Autodesk Inventor part; units mm, degrees
(part 2 of 2)
  line L943 (178.544, 73.9331) -> (164.545, 73.9331)
  line L944 (145.495, 73.9331) -> (145.495, 72.9326)
  line L945 (145.495, 72.9326) -> (144.694, 72.9326)
  line L946 (144.694, 72.9326) -> (144.694, 69.8334)
  line L947 (144.694, 69.8334) -> (145.495, 69.8334)
  line L948 (145.495, 69.8334) -> (145.495, 64.0334)
  line L949 (145.495, 64.0334) -> (144.694, 64.0334)
  line L950 (144.694, 64.0334) -> (144.694, 60.9328)
  line L951 (144.694, 60.9328) -> (145.495, 60.9328)
  line L952 (145.495, 60.9328) -> (145.495, 59.9338)
  line L953 (145.495, 59.9338) -> (159.494, 59.9338)
  line L954 (159.494, 59.9338) -> (159.494, 60.9328)
  line L955 (159.494, 60.9328) -> (160.295, 60.9328)
  line L956 (160.295, 60.9328) -> (160.295, 64.0334)
  line L957 (160.295, 64.0334) -> (159.494, 64.0334)
  line L958 (159.494, 64.0334) -> (159.494, 69.8334)
  line L959 (159.494, 69.8334) -> (160.295, 69.8334)
  line L960 (160.295, 69.8334) -> (160.295, 72.9326)
  line L961 (160.295, 72.9326) -> (159.494, 72.9326)
  line L962 (159.494, 72.9326) -> (159.494, 73.9331)
  line L963 (159.494, 73.9331) -> (145.495, 73.9331)
  line L964 (126.445, 73.9331) -> (126.445, 72.9326)
  line L965 (126.445, 72.9326) -> (125.644, 72.9326)
  line L966 (125.644, 72.9326) -> (125.644, 69.8334)
  line L967 (125.644, 69.8334) -> (126.445, 69.8334)
  line L968 (126.445, 69.8334) -> (126.445, 64.0334)
  line L969 (126.445, 64.0334) -> (125.644, 64.0334)
  line L970 (125.644, 64.0334) -> (125.644, 60.9328)
  line L971 (125.644, 60.9328) -> (126.445, 60.9328)
  line L972 (126.445, 60.9328) -> (126.445, 59.9338)
  line L973 (126.445, 59.9338) -> (140.444, 59.9338)
  line L974 (140.444, 59.9338) -> (140.444, 60.9328)
  line L975 (140.444, 60.9328) -> (141.245, 60.9328)
  line L976 (141.245, 60.9328) -> (141.245, 64.0334)
  line L977 (141.245, 64.0334) -> (140.444, 64.0334)
  line L978 (140.444, 64.0334) -> (140.444, 69.8334)
  line L979 (140.444, 69.8334) -> (141.245, 69.8334)
  line L980 (141.245, 69.8334) -> (141.245, 72.9326)
  line L981 (141.245, 72.9326) -> (140.444, 72.9326)
  line L982 (140.444, 72.9326) -> (140.444, 73.9331)
  line L983 (140.444, 73.9331) -> (126.445, 73.9331)
  line L984 (107.395, 73.9331) -> (107.395, 72.9326)
  line L985 (107.395, 72.9326) -> (106.594, 72.9326)
  line L986 (106.594, 72.9326) -> (106.594, 69.8334)
  line L987 (106.594, 69.8334) -> (107.395, 69.8334)
  line L988 (107.395, 69.8334) -> (107.395, 64.0334)
  line L989 (107.395, 64.0334) -> (106.594, 64.0334)
  line L990 (106.594, 64.0334) -> (106.594, 60.9328)
  line L991 (106.594, 60.9328) -> (107.395, 60.9328)
  line L992 (107.395, 60.9328) -> (107.395, 59.9338)
  line L993 (107.395, 59.9338) -> (121.394, 59.9338)
  line L994 (121.394, 59.9338) -> (121.394, 60.9328)
  line L995 (121.394, 60.9328) -> (122.195, 60.9328)
  line L996 (122.195, 60.9328) -> (122.195, 64.0334)
  line L997 (122.195, 64.0334) -> (121.394, 64.0334)
  line L998 (121.394, 64.0334) -> (121.394, 69.8334)
  line L999 (121.394, 69.8334) -> (122.195, 69.8334)
  line L1000 (122.195, 69.8334) -> (122.195, 72.9326)
  line L1001 (122.195, 72.9326) -> (121.394, 72.9326)
  line L1002 (121.394, 72.9326) -> (121.394, 73.9331)
  line L1003 (121.394, 73.9331) -> (107.395, 73.9331)
  line L1004 (88.3447, 73.9331) -> (88.3447, 72.9326)
  line L1005 (88.3447, 72.9326) -> (87.5439, 72.9326)
  line L1006 (87.5439, 72.9326) -> (87.5439, 69.8334)
  line L1007 (87.5439, 69.8334) -> (88.3447, 69.8334)
  line L1008 (88.3447, 69.8334) -> (88.3447, 64.0334)
  line L1009 (88.3447, 64.0334) -> (87.5439, 64.0334)
  line L1010 (87.5439, 64.0334) -> (87.5439, 60.9328)
  line L1011 (87.5439, 60.9328) -> (88.3447, 60.9328)
  line L1012 (88.3447, 60.9328) -> (88.3447, 59.9338)
  line L1013 (88.3447, 59.9338) -> (102.344, 59.9338)
  line L1014 (102.344, 59.9338) -> (102.344, 60.9328)
  line L1015 (102.344, 60.9328) -> (103.145, 60.9328)
  line L1016 (103.145, 60.9328) -> (103.145, 64.0334)
  line L1017 (103.145, 64.0334) -> (102.344, 64.0334)
  line L1018 (102.344, 64.0334) -> (102.344, 69.8334)
  line L1019 (102.344, 69.8334) -> (103.145, 69.8334)
  line L1020 (103.145, 69.8334) -> (103.145, 72.9326)
  line L1021 (103.145, 72.9326) -> (102.344, 72.9326)
  line L1022 (102.344, 72.9326) -> (102.344, 73.9331)
  line L1023 (102.344, 73.9331) -> (88.3447, 73.9331)
  line L1024 (69.2947, 73.9331) -> (69.2947, 72.9326)
  line L1025 (69.2947, 72.9326) -> (68.4939, 72.9326)
  line L1026 (68.4939, 72.9326) -> (68.4939, 69.8334)
  line L1027 (68.4939, 69.8334) -> (69.2947, 69.8334)
  line L1028 (69.2947, 69.8334) -> (69.2947, 64.0334)
  line L1029 (69.2947, 64.0334) -> (68.4939, 64.0334)
  line L1030 (68.4939, 64.0334) -> (68.4939, 60.9328)
  line L1031 (68.4939, 60.9328) -> (69.2947, 60.9328)
  line L1032 (69.2947, 60.9328) -> (69.2947, 59.9338)
  line L1033 (69.2947, 59.9338) -> (83.294, 59.9338)
  line L1034 (83.294, 59.9338) -> (83.294, 60.9328)
  line L1035 (83.294, 60.9328) -> (84.0948, 60.9328)
  line L1036 (84.0948, 60.9328) -> (84.0948, 64.0334)
  line L1037 (84.0948, 64.0334) -> (83.294, 64.0334)
  line L1038 (83.294, 64.0334) -> (83.294, 69.8334)
  line L1039 (83.294, 69.8334) -> (84.0948, 69.8334)
  line L1040 (84.0948, 69.8334) -> (84.0948, 72.9326)
  line L1041 (84.0948, 72.9326) -> (83.294, 72.9326)
  line L1042 (83.294, 72.9326) -> (83.294, 73.9331)
  line L1043 (83.294, 73.9331) -> (69.2947, 73.9331)
  line L1044 (50.2447, 73.9331) -> (50.2447, 72.9326)
  line L1045 (50.2447, 72.9326) -> (49.4439, 72.9326)
  line L1046 (49.4439, 72.9326) -> (49.4439, 69.8334)
  line L1047 (49.4439, 69.8334) -> (50.2447, 69.8334)
  line L1048 (50.2447, 69.8334) -> (50.2447, 64.0334)
  line L1049 (50.2447, 64.0334) -> (49.4439, 64.0334)
  line L1050 (49.4439, 64.0334) -> (49.4439, 60.9328)
  line L1051 (49.4439, 60.9328) -> (50.2447, 60.9328)
  line L1052 (50.2447, 60.9328) -> (50.2447, 59.9338)
  line L1053 (50.2447, 59.9338) -> (64.244, 59.9338)
  line L1054 (64.244, 59.9338) -> (64.244, 60.9328)
  line L1055 (64.244, 60.9328) -> (65.0448, 60.9328)
  line L1056 (65.0448, 60.9328) -> (65.0448, 64.0334)
  line L1057 (65.0448, 64.0334) -> (64.244, 64.0334)
  line L1058 (64.244, 64.0334) -> (64.244, 69.8334)
  line L1059 (64.244, 69.8334) -> (65.0448, 69.8334)
  line L1060 (65.0448, 69.8334) -> (65.0448, 72.9326)
  line L1061 (65.0448, 72.9326) -> (64.244, 72.9326)
  line L1062 (64.244, 72.9326) -> (64.244, 73.9331)
  line L1063 (64.244, 73.9331) -> (50.2447, 73.9331)
  line L1064 (31.1947, 73.9331) -> (31.1947, 72.9326)
  line L1065 (31.1947, 72.9326) -> (30.394, 72.9326)
  line L1066 (30.394, 72.9326) -> (30.394, 69.8334)
  line L1067 (30.394, 69.8334) -> (31.1947, 69.8334)
  line L1068 (31.1947, 69.8334) -> (31.1947, 64.0334)
  line L1069 (31.1947, 64.0334) -> (30.394, 64.0334)
  line L1070 (30.394, 64.0334) -> (30.394, 60.9328)
  line L1071 (30.394, 60.9328) -> (31.1947, 60.9328)
  line L1072 (31.1947, 60.9328) -> (31.1947, 59.9338)
  line L1073 (31.1947, 59.9338) -> (45.194, 59.9338)
  line L1074 (45.194, 59.9338) -> (45.194, 60.9328)
  line L1075 (45.194, 60.9328) -> (45.9948, 60.9328)
  line L1076 (45.9948, 60.9328) -> (45.9948, 64.0334)
  line L1077 (45.9948, 64.0334) -> (45.194, 64.0334)
  line L1078 (45.194, 64.0334) -> (45.194, 69.8334)
  line L1079 (45.194, 69.8334) -> (45.9948, 69.8334)
  line L1080 (45.9948, 69.8334) -> (45.9948, 72.9326)
  line L1081 (45.9948, 72.9326) -> (45.194, 72.9326)
  line L1082 (45.194, 72.9326) -> (45.194, 73.9331)
  line L1083 (45.194, 73.9331) -> (31.1947, 73.9331)
  line L1084 (7.3822, 73.9331) -> (7.3822, 72.9326)
  line L1085 (7.3822, 72.9326) -> (6.5815, 72.9326)
  line L1086 (6.5815, 72.9326) -> (6.5815, 69.8334)
  line L1087 (6.5815, 69.8334) -> (7.3822, 69.8334)
  line L1088 (7.3822, 69.8334) -> (7.3822, 64.0334)
  line L1089 (7.3822, 64.0334) -> (6.5815, 64.0334)
  line L1090 (6.5815, 64.0334) -> (6.5815, 60.9328)
  line L1091 (6.5815, 60.9328) -> (7.3822, 60.9328)
  line L1092 (7.3822, 60.9328) -> (7.3822, 59.9338)
  line L1093 (7.3822, 59.9338) -> (21.3817, 59.9338)
  line L1094 (21.3817, 59.9338) -> (21.3817, 60.9328)
  line L1095 (21.3817, 60.9328) -> (22.1809, 60.9328)
  line L1096 (22.1809, 60.9328) -> (22.1809, 64.0334)
  line L1097 (22.1809, 64.0334) -> (21.3817, 64.0334)
  line L1098 (21.3817, 64.0334) -> (21.3817, 69.8334)
  line L1099 (21.3817, 69.8334) -> (22.1809, 69.8334)
  line L1100 (22.1809, 69.8334) -> (22.1809, 72.9326)
  line L1101 (22.1809, 72.9326) -> (21.3817, 72.9326)
  line L1102 (21.3817, 72.9326) -> (21.3817, 73.9331)
  line L1103 (21.3817, 73.9331) -> (7.3822, 73.9331)
  line L1104 (259.795, 92.9831) -> (259.795, 91.9826)
  line L1105 (259.795, 91.9826) -> (258.994, 91.9826)
  line L1106 (258.994, 91.9826) -> (258.994, 88.8834)
  line L1107 (258.994, 88.8834) -> (259.795, 88.8834)
  line L1108 (259.795, 88.8834) -> (259.795, 88.2826)
  line L1109 (259.795, 88.2826) -> (258.269, 88.2826)
  line L1110 (258.269, 88.2826) -> (258.269, 91.5127)
  line L1111 (258.269, 91.5127) -> (256.544, 91.5127)
  line L1112 (256.544, 91.5127) -> (256.544, 92.4348)
  line L1113 (256.544, 92.4348) -> (253.243, 92.4348)
  line L1114 (253.243, 92.4348) -> (253.243, 91.5127)
  line L1115 (253.243, 91.5127) -> (251.52, 91.5127)
  line L1116 (251.52, 91.5127) -> (251.52, 88.2826)
  line L1117 (251.52, 88.2826) -> (250.694, 88.2826)
  line L1118 (250.694, 88.2826) -> (250.694, 85.4837)
  line L1119 (250.694, 85.4837) -> (251.52, 85.4837)
  line L1120 (251.52, 85.4837) -> (251.52, 79.2138)
  line L1121 (251.52, 79.2138) -> (253.243, 79.2138)
  line L1122 (253.243, 79.2138) -> (253.243, 78.2327)
  line L1123 (253.243, 78.2327) -> (256.544, 78.2327)
  line L1124 (256.544, 78.2327) -> (256.544, 79.2138)
  line L1125 (256.544, 79.2138) -> (258.269, 79.2138)
  line L1126 (258.269, 79.2138) -> (258.269, 83.6828)
  line L1127 (258.269, 83.6828) -> (259.795, 83.6828)
  line L1128 (259.795, 83.6828) -> (259.795, 83.0834)
  line L1129 (259.795, 83.0834) -> (258.994, 83.0834)
  line L1130 (258.994, 83.0834) -> (258.994, 79.9828)
  line L1131 (258.994, 79.9828) -> (259.795, 79.9828)
  line L1132 (259.795, 79.9828) -> (259.795, 78.9838)
  line L1133 (259.795, 78.9838) -> (273.794, 78.9838)
  line L1134 (273.794, 78.9838) -> (273.794, 79.9828)
  line L1135 (273.794, 79.9828) -> (274.595, 79.9828)
  line L1136 (274.595, 79.9828) -> (274.595, 83.0834)
  line L1137 (274.595, 83.0834) -> (273.794, 83.0834)
  line L1138 (273.794, 83.0834) -> (273.794, 83.6828)
  line L1139 (273.794, 83.6828) -> (275.32, 83.6828)
  line L1140 (275.32, 83.6828) -> (275.32, 79.2138)
  line L1141 (275.32, 79.2138) -> (277.045, 79.2138)
  line L1142 (277.045, 79.2138) -> (277.045, 78.2327)
  line L1143 (277.045, 78.2327) -> (280.344, 78.2327)
  line L1144 (280.344, 78.2327) -> (280.344, 79.2138)
  line L1145 (280.344, 79.2138) -> (282.069, 79.2138)
  line L1146 (282.069, 79.2138) -> (282.069, 85.4837)
  line L1147 (282.069, 85.4837) -> (282.895, 85.4837)
  line L1148 (282.895, 85.4837) -> (282.895, 88.2826)
  line L1149 (282.895, 88.2826) -> (282.069, 88.2826)
  line L1150 (282.069, 88.2826) -> (282.069, 91.5127)
  line L1151 (282.069, 91.5127) -> (280.344, 91.5127)
  line L1152 (280.344, 91.5127) -> (280.344, 92.4348)
  line L1153 (280.344, 92.4348) -> (277.045, 92.4348)
  line L1154 (277.045, 92.4348) -> (277.045, 91.5127)
  line L1155 (277.045, 91.5127) -> (275.32, 91.5127)
  line L1156 (275.32, 91.5127) -> (275.32, 88.2826)
  line L1157 (275.32, 88.2826) -> (273.794, 88.2826)
  line L1158 (273.794, 88.2826) -> (273.794, 88.8834)
  line L1159 (273.794, 88.8834) -> (274.595, 88.8834)
  line L1160 (274.595, 88.8834) -> (274.595, 91.9826)
  line L1161 (274.595, 91.9826) -> (273.794, 91.9826)
  line L1162 (273.794, 91.9826) -> (273.794, 92.9831)
  line L1163 (273.794, 92.9831) -> (259.795, 92.9831)
  line L1164 (231.22, 92.9831) -> (231.22, 91.9826)
  line L1165 (231.22, 91.9826) -> (230.419, 91.9826)
  line L1166 (230.419, 91.9826) -> (230.419, 88.8834)
  line L1167 (230.419, 88.8834) -> (231.22, 88.8834)
  line L1168 (231.22, 88.8834) -> (231.22, 83.0834)
  line L1169 (231.22, 83.0834) -> (230.419, 83.0834)
  line L1170 (230.419, 83.0834) -> (230.419, 79.9828)
  line L1171 (230.419, 79.9828) -> (231.22, 79.9828)
  line L1172 (231.22, 79.9828) -> (231.22, 78.9838)
  line L1173 (231.22, 78.9838) -> (245.219, 78.9838)
  line L1174 (245.219, 78.9838) -> (245.219, 79.9828)
  line L1175 (245.219, 79.9828) -> (246.02, 79.9828)
  line L1176 (246.02, 79.9828) -> (246.02, 83.0834)
  line L1177 (246.02, 83.0834) -> (245.219, 83.0834)
  line L1178 (245.219, 83.0834) -> (245.219, 88.8834)
  line L1179 (245.219, 88.8834) -> (246.02, 88.8834)
  line L1180 (246.02, 88.8834) -> (246.02, 91.9826)
  line L1181 (246.02, 91.9826) -> (245.219, 91.9826)
  line L1182 (245.219, 91.9826) -> (245.219, 92.9831)
  line L1183 (245.219, 92.9831) -> (231.22, 92.9831)
  line L1184 (212.17, 92.9831) -> (212.17, 91.9826)
  line L1185 (212.17, 91.9826) -> (211.369, 91.9826)
  line L1186 (211.369, 91.9826) -> (211.369, 88.8834)
  line L1187 (211.369, 88.8834) -> (212.17, 88.8834)
  line L1188 (212.17, 88.8834) -> (212.17, 83.0834)
  line L1189 (212.17, 83.0834) -> (211.369, 83.0834)
  line L1190 (211.369, 83.0834) -> (211.369, 79.9828)
  line L1191 (211.369, 79.9828) -> (212.17, 79.9828)
  line L1192 (212.17, 79.9828) -> (212.17, 78.9838)
  line L1193 (212.17, 78.9838) -> (226.169, 78.9838)
  line L1194 (226.169, 78.9838) -> (226.169, 79.9828)
  line L1195 (226.169, 79.9828) -> (226.97, 79.9828)
  line L1196 (226.97, 79.9828) -> (226.97, 83.0834)
  line L1197 (226.97, 83.0834) -> (226.169, 83.0834)
  line L1198 (226.169, 83.0834) -> (226.169, 88.8834)
  line L1199 (226.169, 88.8834) -> (226.97, 88.8834)
  line L1200 (226.97, 88.8834) -> (226.97, 91.9826)
  line L1201 (226.97, 91.9826) -> (226.169, 91.9826)
  line L1202 (226.169, 91.9826) -> (226.169, 92.9831)
  line L1203 (226.169, 92.9831) -> (212.17, 92.9831)
  line L1204 (193.12, 92.9831) -> (193.12, 91.9826)
  line L1205 (193.12, 91.9826) -> (192.319, 91.9826)
  line L1206 (192.319, 91.9826) -> (192.319, 88.8834)
  line L1207 (192.319, 88.8834) -> (193.12, 88.8834)
  line L1208 (193.12, 88.8834) -> (193.12, 83.0834)
  line L1209 (193.12, 83.0834) -> (192.319, 83.0834)
  line L1210 (192.319, 83.0834) -> (192.319, 79.9828)
  line L1211 (192.319, 79.9828) -> (193.12, 79.9828)
  line L1212 (193.12, 79.9828) -> (193.12, 78.9838)
  line L1213 (193.12, 78.9838) -> (207.119, 78.9838)
  line L1214 (207.119, 78.9838) -> (207.119, 79.9828)
  line L1215 (207.119, 79.9828) -> (207.92, 79.9828)
  line L1216 (207.92, 79.9828) -> (207.92, 83.0834)
  line L1217 (207.92, 83.0834) -> (207.119, 83.0834)
  line L1218 (207.119, 83.0834) -> (207.119, 88.8834)
  line L1219 (207.119, 88.8834) -> (207.92, 88.8834)
  line L1220 (207.92, 88.8834) -> (207.92, 91.9826)
  line L1221 (207.92, 91.9826) -> (207.119, 91.9826)
  line L1222 (207.119, 91.9826) -> (207.119, 92.9831)
  line L1223 (207.119, 92.9831) -> (193.12, 92.9831)
  line L1224 (174.07, 92.9831) -> (174.07, 91.9826)
  line L1225 (174.07, 91.9826) -> (173.269, 91.9826)
  line L1226 (173.269, 91.9826) -> (173.269, 88.8834)
  line L1227 (173.269, 88.8834) -> (174.07, 88.8834)
  line L1228 (174.07, 88.8834) -> (174.07, 83.0834)
  line L1229 (174.07, 83.0834) -> (173.269, 83.0834)
  line L1230 (173.269, 83.0834) -> (173.269, 79.9828)
  line L1231 (173.269, 79.9828) -> (174.07, 79.9828)
  line L1232 (174.07, 79.9828) -> (174.07, 78.9838)
  line L1233 (174.07, 78.9838) -> (188.069, 78.9838)
  line L1234 (188.069, 78.9838) -> (188.069, 79.9828)
  line L1235 (188.069, 79.9828) -> (188.87, 79.9828)
  line L1236 (188.87, 79.9828) -> (188.87, 83.0834)
  line L1237 (188.87, 83.0834) -> (188.069, 83.0834)
  line L1238 (188.069, 83.0834) -> (188.069, 88.8834)
  line L1239 (188.069, 88.8834) -> (188.87, 88.8834)
  line L1240 (188.87, 88.8834) -> (188.87, 91.9826)
  line L1241 (188.87, 91.9826) -> (188.069, 91.9826)
  line L1242 (188.069, 91.9826) -> (188.069, 92.9831)
  line L1243 (188.069, 92.9831) -> (174.07, 92.9831)
  line L1244 (155.02, 92.9831) -> (155.02, 91.9826)
  line L1245 (155.02, 91.9826) -> (154.219, 91.9826)
  line L1246 (154.219, 91.9826) -> (154.219, 88.8834)
  line L1247 (154.219, 88.8834) -> (155.02, 88.8834)
  line L1248 (155.02, 88.8834) -> (155.02, 83.0834)
  line L1249 (155.02, 83.0834) -> (154.219, 83.0834)
  line L1250 (154.219, 83.0834) -> (154.219, 79.9828)
  line L1251 (154.219, 79.9828) -> (155.02, 79.9828)
  line L1252 (155.02, 79.9828) -> (155.02, 78.9838)
  line L1253 (155.02, 78.9838) -> (169.019, 78.9838)
  line L1254 (169.019, 78.9838) -> (169.019, 79.9828)
  line L1255 (169.019, 79.9828) -> (169.82, 79.9828)
  line L1256 (169.82, 79.9828) -> (169.82, 83.0834)
  line L1257 (169.82, 83.0834) -> (169.019, 83.0834)
  line L1258 (169.019, 83.0834) -> (169.019, 88.8834)
  line L1259 (169.019, 88.8834) -> (169.82, 88.8834)
  line L1260 (169.82, 88.8834) -> (169.82, 91.9826)
  line L1261 (169.82, 91.9826) -> (169.019, 91.9826)
  line L1262 (169.019, 91.9826) -> (169.019, 92.9831)
  line L1263 (169.019, 92.9831) -> (155.02, 92.9831)
  line L1264 (135.97, 92.9831) -> (135.97, 91.9826)
  line L1265 (135.97, 91.9826) -> (135.169, 91.9826)
  line L1266 (135.169, 91.9826) -> (135.169, 88.8834)
  line L1267 (135.169, 88.8834) -> (135.97, 88.8834)
  line L1268 (135.97, 88.8834) -> (135.97, 83.0834)
  line L1269 (135.97, 83.0834) -> (135.169, 83.0834)
  line L1270 (135.169, 83.0834) -> (135.169, 79.9828)
  line L1271 (135.169, 79.9828) -> (135.97, 79.9828)
  line L1272 (135.97, 79.9828) -> (135.97, 78.9838)
  line L1273 (135.97, 78.9838) -> (149.969, 78.9838)
  line L1274 (149.969, 78.9838) -> (149.969, 79.9828)
  line L1275 (149.969, 79.9828) -> (150.77, 79.9828)
  line L1276 (150.77, 79.9828) -> (150.77, 83.0834)
  line L1277 (150.77, 83.0834) -> (149.969, 83.0834)
  line L1278 (149.969, 83.0834) -> (149.969, 88.8834)
  line L1279 (149.969, 88.8834) -> (150.77, 88.8834)
  line L1280 (150.77, 88.8834) -> (150.77, 91.9826)
  line L1281 (150.77, 91.9826) -> (149.969, 91.9826)
  line L1282 (149.969, 91.9826) -> (149.969, 92.9831)
  line L1283 (149.969, 92.9831) -> (135.97, 92.9831)
  line L1284 (116.918, 92.9831) -> (116.918, 91.9826)
  line L1285 (116.918, 91.9826) -> (116.119, 91.9826)
  line L1286 (116.119, 91.9826) -> (116.119, 88.8834)
  line L1287 (116.119, 88.8834) -> (116.918, 88.8834)
  line L1288 (116.918, 88.8834) -> (116.918, 83.0834)
  line L1289 (116.918, 83.0834) -> (116.119, 83.0834)
  line L1290 (116.119, 83.0834) -> (116.119, 79.9828)
  line L1291 (116.119, 79.9828) -> (116.918, 79.9828)
  line L1292 (116.918, 79.9828) -> (116.918, 78.9838)
  line L1293 (116.918, 78.9838) -> (130.919, 78.9838)
  line L1294 (130.919, 78.9838) -> (130.919, 79.9828)
  line L1295 (130.919, 79.9828) -> (131.72, 79.9828)
  line L1296 (131.72, 79.9828) -> (131.72, 83.0834)
  line L1297 (131.72, 83.0834) -> (130.919, 83.0834)
  line L1298 (130.919, 83.0834) -> (130.919, 88.8834)
  line L1299 (130.919, 88.8834) -> (131.72, 88.8834)
  line L1300 (131.72, 88.8834) -> (131.72, 91.9826)
  line L1301 (131.72, 91.9826) -> (130.919, 91.9826)
  line L1302 (130.919, 91.9826) -> (130.919, 92.9831)
  line L1303 (130.919, 92.9831) -> (116.918, 92.9831)
  line L1304 (97.8683, 92.9831) -> (97.8683, 91.9826)
  line L1305 (97.8683, 91.9826) -> (97.0689, 91.9826)
  line L1306 (97.0689, 91.9826) -> (97.0689, 88.8834)
  line L1307 (97.0689, 88.8834) -> (97.8683, 88.8834)
  line L1308 (97.8683, 88.8834) -> (97.8683, 83.0834)
  line L1309 (97.8683, 83.0834) -> (97.0689, 83.0834)
  line L1310 (97.0689, 83.0834) -> (97.0689, 79.9828)
  line L1311 (97.0689, 79.9828) -> (97.8683, 79.9828)
  line L1312 (97.8683, 79.9828) -> (97.8683, 78.9838)
  line L1313 (97.8683, 78.9838) -> (111.869, 78.9838)
  line L1314 (111.869, 78.9838) -> (111.869, 79.9828)
  line L1315 (111.869, 79.9828) -> (112.668, 79.9828)
  line L1316 (112.668, 79.9828) -> (112.668, 83.0834)
  line L1317 (112.668, 83.0834) -> (111.869, 83.0834)
  line L1318 (111.869, 83.0834) -> (111.869, 88.8834)
  line L1319 (111.869, 88.8834) -> (112.668, 88.8834)
  line L1320 (112.668, 88.8834) -> (112.668, 91.9826)
  line L1321 (112.668, 91.9826) -> (111.869, 91.9826)
  line L1322 (111.869, 91.9826) -> (111.869, 92.9831)
  line L1323 (111.869, 92.9831) -> (97.8683, 92.9831)
  line L1324 (78.8197, 92.9831) -> (78.8197, 91.9826)
  line L1325 (78.8197, 91.9826) -> (78.0189, 91.9826)
  line L1326 (78.0189, 91.9826) -> (78.0189, 88.8834)
  line L1327 (78.0189, 88.8834) -> (78.8197, 88.8834)
  line L1328 (78.8197, 88.8834) -> (78.8197, 83.0834)
  line L1329 (78.8197, 83.0834) -> (78.0189, 83.0834)
  line L1330 (78.0189, 83.0834) -> (78.0189, 79.9828)
  line L1331 (78.0189, 79.9828) -> (78.8197, 79.9828)
  line L1332 (78.8197, 79.9828) -> (78.8197, 78.9838)
  line L1333 (78.8197, 78.9838) -> (92.819, 78.9838)
  line L1334 (92.819, 78.9838) -> (92.819, 79.9828)
  line L1335 (92.819, 79.9828) -> (93.6184, 79.9828)
  line L1336 (93.6184, 79.9828) -> (93.6184, 83.0834)
  line L1337 (93.6184, 83.0834) -> (92.819, 83.0834)
  line L1338 (92.819, 83.0834) -> (92.819, 88.8834)
  line L1339 (92.819, 88.8834) -> (93.6184, 88.8834)
  line L1340 (93.6184, 88.8834) -> (93.6184, 91.9826)
  line L1341 (93.6184, 91.9826) -> (92.819, 91.9826)
  line L1342 (92.819, 91.9826) -> (92.819, 92.9831)
  line L1343 (92.819, 92.9831) -> (78.8197, 92.9831)
  line L1344 (59.7697, 92.9831) -> (59.7697, 91.9826)
  line L1345 (59.7697, 91.9826) -> (58.9689, 91.9826)
  line L1346 (58.9689, 91.9826) -> (58.9689, 88.8834)
  line L1347 (58.9689, 88.8834) -> (59.7697, 88.8834)
  line L1348 (59.7697, 88.8834) -> (59.7697, 83.0834)
  line L1349 (59.7697, 83.0834) -> (58.9689, 83.0834)
  line L1350 (58.9689, 83.0834) -> (58.9689, 79.9828)
  line L1351 (58.9689, 79.9828) -> (59.7697, 79.9828)
  line L1352 (59.7697, 79.9828) -> (59.7697, 78.9838)
  line L1353 (59.7697, 78.9838) -> (73.769, 78.9838)
  line L1354 (73.769, 78.9838) -> (73.769, 79.9828)
  line L1355 (73.769, 79.9828) -> (74.5698, 79.9828)
  line L1356 (74.5698, 79.9828) -> (74.5698, 83.0834)
  line L1357 (74.5698, 83.0834) -> (73.769, 83.0834)
  line L1358 (73.769, 83.0834) -> (73.769, 88.8834)
  line L1359 (73.769, 88.8834) -> (74.5698, 88.8834)
  line L1360 (74.5698, 88.8834) -> (74.5698, 91.9826)
  line L1361 (74.5698, 91.9826) -> (73.769, 91.9826)
  line L1362 (73.769, 91.9826) -> (73.769, 92.9831)
  line L1363 (73.769, 92.9831) -> (59.7697, 92.9831)
  line L1364 (40.7197, 92.9831) -> (40.7197, 91.9826)
  line L1365 (40.7197, 91.9826) -> (39.9189, 91.9826)
  line L1366 (39.9189, 91.9826) -> (39.9189, 88.8834)
  line L1367 (39.9189, 88.8834) -> (40.7197, 88.8834)
  line L1368 (40.7197, 88.8834) -> (40.7197, 83.0834)
  line L1369 (40.7197, 83.0834) -> (39.9189, 83.0834)
  line L1370 (39.9189, 83.0834) -> (39.9189, 79.9828)
  line L1371 (39.9189, 79.9828) -> (40.7197, 79.9828)
  line L1372 (40.7197, 79.9828) -> (40.7197, 78.9838)
  line L1373 (40.7197, 78.9838) -> (54.719, 78.9838)
  line L1374 (54.719, 78.9838) -> (54.719, 79.9828)
  line L1375 (54.719, 79.9828) -> (55.5198, 79.9828)
  line L1376 (55.5198, 79.9828) -> (55.5198, 83.0834)
  line L1377 (55.5198, 83.0834) -> (54.719, 83.0834)
  line L1378 (54.719, 83.0834) -> (54.719, 88.8834)
  line L1379 (54.719, 88.8834) -> (55.5198, 88.8834)
  line L1380 (55.5198, 88.8834) -> (55.5198, 91.9826)
  line L1381 (55.5198, 91.9826) -> (54.719, 91.9826)
  line L1382 (54.719, 91.9826) -> (54.719, 92.9831)
  line L1383 (54.719, 92.9831) -> (40.7197, 92.9831)
  line L1384 (21.6697, 92.9831) -> (21.6697, 91.9826)
  line L1385 (21.6697, 91.9826) -> (20.869, 91.9826)
  line L1386 (20.869, 91.9826) -> (20.869, 88.8834)
  line L1387 (20.869, 88.8834) -> (21.6697, 88.8834)
  line L1388 (21.6697, 88.8834) -> (21.6697, 83.0834)
  line L1389 (21.6697, 83.0834) -> (20.869, 83.0834)
  line L1390 (20.869, 83.0834) -> (20.869, 79.9828)
  line L1391 (20.869, 79.9828) -> (21.6697, 79.9828)
  line L1392 (21.6697, 79.9828) -> (21.6697, 78.9838)
  line L1393 (21.6697, 78.9838) -> (35.669, 78.9838)
  line L1394 (35.669, 78.9838) -> (35.669, 79.9828)
  line L1395 (35.669, 79.9828) -> (36.4698, 79.9828)
  line L1396 (36.4698, 79.9828) -> (36.4698, 83.0834)
  line L1397 (36.4698, 83.0834) -> (35.669, 83.0834)
  line L1398 (35.669, 83.0834) -> (35.669, 88.8834)
  line L1399 (35.669, 88.8834) -> (36.4698, 88.8834)
  line L1400 (36.4698, 88.8834) -> (36.4698, 91.9826)
  line L1401 (36.4698, 91.9826) -> (35.669, 91.9826)
  line L1402 (35.669, 91.9826) -> (35.669, 92.9831)
  line L1403 (35.669, 92.9831) -> (21.6697, 92.9831)
  line L1404 (2.6197, 92.9831) -> (2.6197, 91.9826)
  line L1405 (2.6197, 91.9826) -> (1.819, 91.9826)
  line L1406 (1.819, 91.9826) -> (1.819, 88.8834)
  line L1407 (1.819, 88.8834) -> (2.6197, 88.8834)
  line L1408 (2.6197, 88.8834) -> (2.6197, 83.0834)
  line L1409 (2.6197, 83.0834) -> (1.819, 83.0834)
  line L1410 (1.819, 83.0834) -> (1.819, 79.9828)
  line L1411 (1.819, 79.9828) -> (2.6197, 79.9828)
  line L1412 (2.6197, 79.9828) -> (2.6197, 78.9838)
  line L1413 (2.6197, 78.9838) -> (16.6192, 78.9838)
  line L1414 (16.6192, 78.9838) -> (16.6192, 79.9828)
  line L1415 (16.6192, 79.9828) -> (17.4198, 79.9828)
  line L1416 (17.4198, 79.9828) -> (17.4198, 83.0834)
  line L1417 (17.4198, 83.0834) -> (16.6192, 83.0834)
  line L1418 (16.6192, 83.0834) -> (16.6192, 88.8834)
  line L1419 (16.6192, 88.8834) -> (17.4198, 88.8834)
  line L1420 (17.4198, 88.8834) -> (17.4198, 91.9826)
  line L1421 (17.4198, 91.9826) -> (16.6192, 91.9826)
  line L1422 (16.6192, 91.9826) -> (16.6192, 92.9831)
  line L1423 (16.6192, 92.9831) -> (2.6197, 92.9831)
  point P0 (0, 0)
  point P1 (0.0951, 0.2577)
  constraints: 2848 end point
extrude "Extrusion1" add sketch "Sketch1" along normal blind 5.08
body "Solid1"
